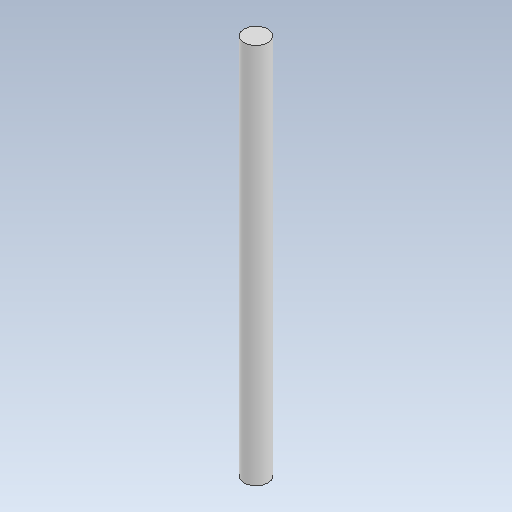
# Autodesk Inventor part: roller_shaft
Saved by Autodesk Inventor 2021 (Build 250183000, 183)
## iProperties
Created: 2022-10-17
Part Number: roller_shaft
Material: Generic
Document SubType Name: Modeling
Designer: Jonathan
Density: 1 g/cm^3
Appearance: Default
Author: Jonathan
Autodesk Inventor part; units mm, degrees
ref_plane "YZ Plane" through (0, 0, 0) normal (1, 0, 0) x (0, 1, 0)
ref_plane "XZ Plane" through (0, 0, 0) normal (0, 1, 0) x (-1, 0, 0)
ref_plane "XY Plane" through (0, 0, 0) normal (0, 0, 1) x (1, 0, 0)
sketch "Sketch1" plane through (0, 0, 0) normal (0, 1, 0) x (-1, 0, 0)
  circle A0 centre (0, 0) radius 1.5875
  dimension "d0" = 3.175
  constraints: 1 centre point, 1 coincident
  measures "d0" diameter of A0
extrude "Extrusion1" add sketch "Sketch1" along normal mid plane 50.8
equation "\"d0\" = roller_shaft_d"
equation "\"d1\" = roller_shaft_l"
equation "\"roller_shaft_d\" = 3.175"
equation "\"roller_shaft_l\" = 50.8"
body "Solid1"
